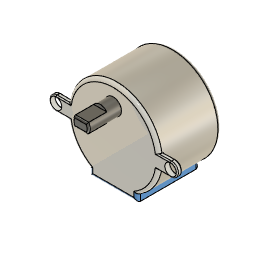
Decombinator v44 (Autodesk Fusion 360 archive; units mm, degrees)
design "small stepper"
Autodesk Fusion 360 part; units mm, degrees
sketch "Sketch1" plane through (0, 0, 0) normal (0, 1, 0) x (1, 0, 0) in component "ELEGOO stepper"
  circle A0 centre (17.5, 0) radius 1.75
  circle A1 centre (0, -8) radius 2.5
  line L0 (0, 0) -> (0, -30.6582) construction
  line L1 (0, 0) -> (-33.3553, 0) construction
  line L2 (0, 0) -> (0, 28) construction
  line L3 (0, 0) -> (32.2921, 0) construction
  line L4 (-7.3, 11.9461) -> (-7.3, 14)
  line L5 (-7.3, 14) -> (7.3, 14)
  line L6 (7.3, 14) -> (7.3, 11.9461)
  line L7 (0, 15.1083) -> (-7.3, 14) construction
  line L8 (17.4702, -2.0998) -> (13.8493, -2.0485)
  line L9 (17.5, 2.1) -> (13.8416, 2.1)
  arc A2 (17.4702, -2.0998) -> (17.5, 2.1) centre (17.5, 0) ccw
  arc A3 (-7.3, 11.9461) -> (7.3, 11.9461) centre (0, 0) ccw
  line L10 (0, -14) -> (-22.5265, -14) construction
  line L11 (-17.4702, -2.0998) -> (-13.8493, -2.0485)
  circle A4 centre (-17.5, 0) radius 1.75
  arc A5 (-17.5, 2.1) -> (-17.4702, -2.0998) centre (-17.5, 0) ccw
  line L12 (-17.5, 2.1) -> (-13.8416, 2.1)
  dimension "d1" = 28
  dimension "d2" = 14.6
  dimension "d4" = 3.5
  dimension "d5" = 17.5
  dimension "d6" = 4.2
  dimension "d7" = 8
  dimension "d8" = 5
  dimension "d9" = 28
  constraint coincident L0.start L1.start
  constraint vertical L0
  constraint perpendicular L0 L1
  constraint coincident A1.centre L0
  constraint perpendicular L1 L2
  constraint horizontal L3
  constraint parallel L4 L6
  constraint coincident A0.centre L3
  constraint concentric A0 A2
  constraint coincident L8.end A3
  constraint tangent L8 A2
  constraint coincident L9.end A3
  constraint horizontal L9
  constraint tangent L9 A2
  constraint coincident L2 L7.start
  constraint horizontal L5
  constraint vertical L4
  constraint midpoint L2 L5
  constraint midpoint A3 L10.start
  constraint tangent A3 L10
  constraint perpendicular L0 L10
  constraint symmetric A0 L0 A4
  constraint symmetric L0 L8.start L11.start
  constraint symmetric L0 L8.end L11.end
  constraint symmetric L0 L9.start A5.start
  constraint symmetric L0 L9.end L12.end
  constraint symmetric L0 A2 A5
  measures "d1" diameter of A3
  measures "d2" distance of L4 L6
  measures "d4" diameter of A0
  measures "d5" distance of A0.centre L2
  measures "d6" diameter of A2
  measures "d7" vertical distance of A1.centre A0.centre
  measures "d8" diameter of A1
  measures "d9" distance of L5 L10
extrude "Extrude1" add sketch "Sketch1" along normal blind 19 contours A1 | L4 L5 L6 A3 in component "ELEGOO stepper"
extrude "Extrude2" add sketch "Sketch1" against normal blind 10 contours A1 in component "ELEGOO stepper"
extrude "Extrude3" add sketch "Sketch1" along normal blind 1.5 contours A3 L11 A5 L12 | L8 L9 A2 A3 in component "ELEGOO stepper"
sketch "Sketch2" plane through (0, -10, 0) normal (0, -1, 0) x (1, 0, 0) in component "ELEGOO stepper"
  line L0 (-4.0846, 9.5) -> (7.5998, 9.5)
  line L1 (-4.0846, 6.5) -> (6.4773, 6.5)
  circle A0 centre (0, 8) radius 2.5
  line L2 (0, 8) -> (11.7837, 8) construction
  dimension "d16" = 3
  constraint horizontal L0
  constraint parallel L0 L1
  constraint coincident A0.centre L2.start
  constraint parallel L0 L2
  measures "d16" distance of L0 L1
extrude "Extrude4" cut sketch "Sketch2" against normal blind 6 contours L0 A0 | L1 A0 in component "ELEGOO stepper"
fillet "Fillet1" radius 0.484 1 faces at (-0.608, -10, 7.5897) in component "ELEGOO stepper"
fillet "Fillet2" radius 1.019 10 edges at (0, 19, 14) (0, 0, 14) (11.661, 0, -7.7474) (-7.3, 0, -12.9731) (7.3, 0, -12.9731) (7.3, 19, -12.9731) (-7.3, 19, -12.9731) (0, 19, -14) (0, 0, -14) (-11.661, 0, -7.7474) in component "ELEGOO stepper"
fillet "Fillet3" radius 0.329 12 edges at (15.155, 0, -2.1) (19.5999, 0, 0.0149) (15.1455, 0, 2.0668) (15.6598, 1.5, 2.0741) (19.5999, 1.5, 0.0149) (15.6708, 1.5, -2.1) (-15.6708, 1.5, -2.1) (-19.5999, 1.5, 0.0149) (-15.6598, 1.5, 2.0741) (-15.6708, 0, -2.1) (-19.5999, 0, 0.0149) (-15.1455, 0, 2.0668) in component "ELEGOO stepper"
form "Form1" [no effect] in component "ELEGOO stepper"
component "ELEGOO stepper" placed x (1, 0, 0) y (0, 1, 0) z (0, 0, 1) at (0, 0, 0)
equation "d5 = ( 35 / 2 ) * 1 mm"
